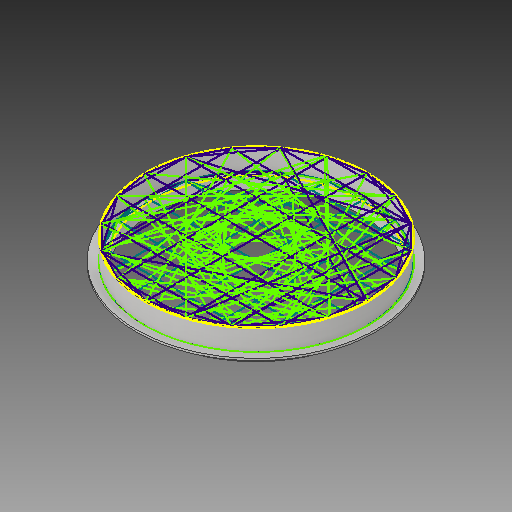
# Autodesk Inventor part: 除沫器
Saved by Autodesk Inventor 2018.2 (Build 222227000, 227)
## iProperties
Created: 2018-07-04
Part Number: 除沫器
Material: 常规
Document SubType Name: Modeling
Designer: Administrator
Density: 1 g/cm^3
Appearance: 默认
Author: Administrator
Autodesk Inventor part; units mm, degrees
ref_plane "YZ Plane" through (0, 0, 0) normal (1, 0, 0) x (0, 1, 0)
ref_plane "XZ Plane" through (0, 0, 0) normal (0, 1, 0) x (-1, 0, 0)
ref_plane "XY Plane" through (0, 0, 0) normal (0, 0, 1) x (1, 0, 0)
sketch "草图1" plane through (0, 0, 0) normal (0, 1, 0) x (-1, 0, 0)
  circle A0 centre (0, 0) radius 575
  circle A1 centre (0, 0) radius 510
  dimension "d0" = 1150
  dimension "d1" = 1020
  constraints: 2 centre point, 2 coincident
  measures "d0" diameter of A0
  measures "d1" diameter of A1
extrude "拉伸1" add sketch "草图1" along normal blind 10
sketch "草图2" plane through (0, 0, 0) normal (0, 1, 0) x (-1, 0, 0)
  circle A0 centre (0, 0) radius 510 projected
surface extrude "拉伸曲面1" sketch "草图2" along normal blind 10 and the other way blind 50 shown no curves A0
thicken "加厚1" operation add thickness 5 both sides no extend neighbours no toward (0.7479816, 0, 0.6637194) faces at (-381.4706, 6.6667, -338.4969) (-381.4706, -30, -338.4969)
sketch "草图3" plane through (0, 10, 0) normal (0, 1, 0) x (1, 0, 0)
  circle A0 centre (0, 0) radius 575 projected
  circle A1 centre (0, 0) radius 536.0493
  constraints: 1 centre point, 1 coincident
surface extrude "拉伸曲面2" sketch "草图3" along normal blind 100 shown no curves A1
thicken "加厚2" operation add thickness 5 both sides no extend neighbours no toward (-0.9991732, 0, -0.0406567) faces at (535.606, 76.6667, 21.794)
sketch "草图4" plane through (0, 110, 0) normal (0, 1, 0) x (1, 0, 0)
  circle A0 centre (0, 0) radius 536.0493 projected
  circle A1 centre (0, 0) radius 531.0493 projected
  line L0 (531.0493, 0) -> (505.0579, -164.1032)
  line L1 (505.0579, -164.1032) -> (429.6279, -312.1429)
  line L2 (429.6279, -312.1429) -> (312.1429, -429.6279)
  line L3 (312.1429, -429.6279) -> (164.1032, -505.0579)
  line L4 (164.1032, -505.0579) -> (0, -531.0493)
  line L5 (0, -531.0493) -> (-164.1032, -505.0579)
  line L6 (-164.1032, -505.0579) -> (-312.1429, -429.6279)
  line L7 (-312.1429, -429.6279) -> (-429.6279, -312.1429)
  line L8 (-429.6279, -312.1429) -> (-505.0579, -164.1032)
  line L9 (-505.0579, -164.1032) -> (-531.0493, 0)
  line L10 (-531.0493, 0) -> (-505.0579, 164.1032)
  line L11 (-505.0579, 164.1032) -> (-429.6279, 312.1429)
  line L12 (-429.6279, 312.1429) -> (-312.1429, 429.6279)
  line L13 (-312.1429, 429.6279) -> (-164.1032, 505.0579)
  line L14 (-164.1032, 505.0579) -> (0, 531.0493)
  line L15 (0, 531.0493) -> (164.1032, 505.0579)
  line L16 (164.1032, 505.0579) -> (312.1429, 429.6279)
  line L17 (312.1429, 429.6279) -> (429.6279, 312.1429)
  line L18 (429.6279, 312.1429) -> (505.0579, 164.1032)
  line L19 (505.0579, 164.1032) -> (531.0493, 0)
  line L20 (-531.0493, 0) -> (531.0493, 0)
  line L21 (-505.0579, 164.1032) -> (-505.0579, -164.1032)
  line L22 (-429.6279, 312.1429) -> (-429.6279, -312.1429)
  line L23 (-312.1429, 429.6279) -> (-312.1429, -429.6279)
  line L24 (-164.1032, 505.0579) -> (-164.1032, -505.0579)
  line L25 (0, 531.0493) -> (0, -531.0493)
  line L26 (164.1032, 505.0579) -> (164.1032, -505.0579)
  line L27 (312.1429, -429.6279) -> (312.1429, 429.6279)
  line L28 (429.6279, 312.1429) -> (429.6279, -312.1429)
  line L29 (505.0579, -164.1032) -> (505.0579, 164.1032)
  line L30 (-164.1032, 505.0579) -> (164.1032, 505.0579)
  line L31 (312.1429, 429.6279) -> (-312.1429, 429.6279)
  line L32 (-429.6279, 312.1429) -> (429.6279, 312.1429)
  line L33 (505.0579, 164.1032) -> (-505.0579, 164.1032)
  line L34 (-505.0579, -164.1032) -> (505.0579, -164.1032)
  line L35 (-429.6279, -312.1429) -> (429.6279, -312.1429)
  line L36 (312.1429, -429.6279) -> (-312.1429, -435.7931)
  line L37 (-164.1032, -505.0579) -> (164.1032, -505.0579)
  line L38 (-312.1429, 429.6279) -> (-505.0579, 164.1032)
  line L39 (-505.0579, -164.1032) -> (-312.1429, -435.7931)
  line L40 (0, -531.0493) -> (-312.1429, -435.7931)
  line L41 (0, -531.0493) -> (312.1429, -429.6279)
  line L42 (312.1429, -429.6279) -> (505.0579, -164.1032)
  line L43 (505.0579, 164.1032) -> (312.1429, 429.6279)
  line L44 (312.1429, 429.6279) -> (0, 531.0493)
  line L45 (531.0493, 0) -> (-312.1429, -435.7931)
  line L46 (-312.1429, 429.6279) -> (531.0493, 0)
  line L47 (312.1429, 429.6279) -> (164.1032, -505.0579)
  line L48 (164.1032, -505.0579) -> (-505.0579, 164.1032)
  line L49 (-505.0579, 164.1032) -> (312.1429, 429.6279)
  line L50 (-429.6279, -312.1429) -> (429.6279, -312.1429)
  line L51 (0, 531.0493) -> (435.7931, -312.1429)
  line L52 (-429.6279, -312.1429) -> (0, 531.0493)
  line L53 (-312.1429, -429.6279) -> (505.0579, -164.1032)
  line L54 (-312.1429, -429.6279) -> (-164.1032, 505.0579)
  line L55 (-164.1032, 505.0579) -> (510.9213, -162.1981)
  line L56 (-505.9804, -165.9401) -> (161.2755, 509.0845)
  line L57 (428.7053, -313.9798) -> (-505.9804, -165.9401)
  line L58 (429.6279, -312.1429) -> (164.1032, 505.0579)
  line L59 (164.1032, -505.0579) -> (-505.0579, 164.1032)
  line L60 (-505.0579, 164.1032) -> (431.533, 318.0064)
  line L61 (164.1032, -505.0579) -> (429.6279, 312.1429)
  line L62 (-429.6279, 312.1429) -> (508.6817, 169.091)
  line L63 (0, -531.0493) -> (-429.6279, 312.1429)
  line L64 (0, -531.0493) -> (505.0579, 164.1032)
  line L65 (311.2203, -431.4647) -> (-536.9596, -5.4607)
  line L66 (164.1032, 505.0579) -> (-531.0493, 0)
  line L67 (163.1807, 503.221) -> (311.2203, -431.4647)
  line L68 (-316.3703, 426.5245) -> (535.9751, 8.9171)
  line L69 (-159.1077, -506.6538) -> (531.0234, 5.2442)
  line L70 (-159.1077, -506.6538) -> (-316.3703, 426.5245)
  line L71 (508.2003, -154.0967) -> (-425.1685, -326.4668)
  line L72 (-174.0458, 501.7184) -> (508.2003, -154.0967)
  line L73 (-174.0458, 501.7184) -> (-423.3795, -320.5669)
  line L74 (-111.947, 217.7208) -> (244.5252, -11.9114)
  line L75 (244.5252, -11.9114) -> (-132.5782, -205.8094)
  line L76 (-132.5782, -205.8094) -> (-111.947, 217.7208)
  line L77 (-210.9866, 63.9755) -> (160.8977, 150.7321)
  line L78 (160.8977, 150.7321) -> (50.0889, -214.7075)
  line L79 (50.0889, -214.7075) -> (-210.9866, 63.9755)
  line L80 (-231.596, -76.5164) -> (49.5329, 238.8263)
  line L81 (49.5329, 238.8263) -> (182.0632, -162.3098)
  line L82 (182.0632, -162.3098) -> (-231.596, -76.5164)
  line L83 (-178.3739, -185.5628) -> (-71.5151, 247.2577)
  line L84 (-71.5151, 247.2577) -> (249.889, -61.6949)
  line L85 (249.889, -61.6949) -> (-178.3739, -185.5628)
  line L86 (-84.545, -232.6889) -> (-159.242, 189.5626)
  line L87 (-159.242, 189.5626) -> (243.787, 43.1263)
  line L88 (243.787, 43.1263) -> (-84.545, -232.6889)
  line L89 (0, -247.9487) -> (-214.7299, 123.9744)
  line L90 (-214.7299, 123.9744) -> (214.7299, 123.9744)
  line L91 (214.7299, 123.9744) -> (0, -247.9487)
  line L92 (79.8324, -233.2057) -> (-241.8782, 47.466)
  line L93 (-241.8782, 47.466) -> (162.0458, 185.7397)
  line L94 (162.0458, 185.7397) -> (79.8324, -233.2057)
  line L95 (218.5126, -161.5306) -> (-249.1459, -108.4722)
  line L96 (-249.1459, -108.4722) -> (30.6333, 270.0028)
  line L97 (30.6333, 270.0028) -> (218.5126, -161.5306)
  point P0 (0, 0)
  point P1 (0, 0)
  point P2 (0, 0)
  point P3 (0, 0)
  constraints: 196 end point, 15 point on line, 13 parallel, 7 coincident, 2 midpoint, 2 perpendicular, 2 point on circle, 1 horizontal, 99 other
sketch "草图5" plane through (0, 10, 0) normal (0, 1, 0) x (1, 0, 0)
  circle A0 centre (0, 0) radius 531.0493 projected
  circle A1 centre (0, 0) radius 505 projected
  circle A2 centre (0, 0) radius 536.0493
  circle A3 centre (0, 0) radius 531.0493
  line L0 (531.0493, 0) -> (505.0579, -164.1032)
  line L1 (505.0579, -164.1032) -> (429.6279, -312.1429)
  line L2 (429.6279, -312.1429) -> (312.1429, -429.6279)
  line L3 (312.1429, -429.6279) -> (164.1032, -505.0579)
  line L4 (164.1032, -505.0579) -> (0, -531.0493)
  line L5 (0, -531.0493) -> (-164.1032, -505.0579)
  line L6 (-164.1032, -505.0579) -> (-312.1429, -429.6279)
  line L7 (-312.1429, -429.6279) -> (-429.6279, -312.1429)
  line L8 (-429.6279, -312.1429) -> (-505.0579, -164.1032)
  line L9 (-505.0579, -164.1032) -> (-531.0493, 0)
  line L10 (-531.0493, 0) -> (-505.0579, 164.1032)
  line L11 (-505.0579, 164.1032) -> (-429.6279, 312.1429)
  line L12 (-429.6279, 312.1429) -> (-312.1429, 429.6279)
  line L13 (-312.1429, 429.6279) -> (-164.1032, 505.0579)
  line L14 (-164.1032, 505.0579) -> (0, 531.0493)
  line L15 (0, 531.0493) -> (164.1032, 505.0579)
  line L16 (164.1032, 505.0579) -> (312.1429, 429.6279)
  line L17 (312.1429, 429.6279) -> (429.6279, 312.1429)
  line L18 (429.6279, 312.1429) -> (505.0579, 164.1032)
  line L19 (505.0579, 164.1032) -> (531.0493, 0)
  line L20 (-531.0493, 0) -> (531.0493, 0)
  line L21 (-505.0579, 164.1032) -> (-505.0579, -164.1032)
  line L22 (-429.6279, 312.1429) -> (-429.6279, -312.1429)
  line L23 (-312.1429, 429.6279) -> (-312.1429, -429.6279)
  line L24 (-164.1032, 505.0579) -> (-164.1032, -505.0579)
  line L25 (0, 531.0493) -> (0, -531.0493)
  line L26 (164.1032, 505.0579) -> (164.1032, -505.0579)
  line L27 (312.1429, -429.6279) -> (312.1429, 429.6279)
  line L28 (429.6279, 312.1429) -> (429.6279, -312.1429)
  line L29 (505.0579, -164.1032) -> (505.0579, 164.1032)
  line L30 (-164.1032, 505.0579) -> (164.1032, 505.0579)
  line L31 (312.1429, 429.6279) -> (-312.1429, 429.6279)
  line L32 (-429.6279, 312.1429) -> (429.6279, 312.1429)
  line L33 (505.0579, 164.1032) -> (-505.0579, 164.1032)
  line L34 (-505.0579, -164.1032) -> (505.0579, -164.1032)
  line L35 (-429.6279, -312.1429) -> (429.6279, -312.1429)
  line L36 (312.1429, -429.6279) -> (-312.1429, -435.7931)
  line L37 (-164.1032, -505.0579) -> (164.1032, -505.0579)
  line L38 (-312.1429, 429.6279) -> (-505.0579, 164.1032)
  line L39 (-505.0579, -164.1032) -> (-312.1429, -435.7931)
  line L40 (0, -531.0493) -> (-312.1429, -435.7931)
  line L41 (0, -531.0493) -> (312.1429, -429.6279)
  line L42 (312.1429, -429.6279) -> (505.0579, -164.1032)
  line L43 (505.0579, 164.1032) -> (312.1429, 429.6279)
  line L44 (312.1429, 429.6279) -> (0, 531.0493)
  line L45 (531.0493, 0) -> (-312.1429, -435.7931)
  line L46 (-312.1429, 429.6279) -> (531.0493, 0)
  line L47 (312.1429, 429.6279) -> (164.1032, -505.0579)
  line L48 (164.1032, -505.0579) -> (-505.0579, 164.1032)
  line L49 (-505.0579, 164.1032) -> (312.1429, 429.6279)
  line L50 (-429.6279, -312.1429) -> (429.6279, -312.1429)
  line L51 (-429.6279, -312.1429) -> (0, 531.0493)
  line L52 (0, 531.0493) -> (435.7931, -312.1429)
  line L53 (-164.1032, 505.0579) -> (510.9213, -162.1981)
  line L54 (-312.1429, -429.6279) -> (-164.1032, 505.0579)
  line L55 (-312.1429, -429.6279) -> (505.0579, -164.1032)
  line L56 (428.7053, -313.9798) -> (-505.9804, -165.9401)
  line L57 (-505.9804, -165.9401) -> (161.2755, 509.0845)
  line L58 (429.6279, -312.1429) -> (164.1032, 505.0579)
  line L59 (-505.0579, 164.1032) -> (431.533, 318.0064)
  line L60 (164.1032, -505.0579) -> (-505.0579, 164.1032)
  line L61 (164.1032, -505.0579) -> (429.6279, 312.1429)
  line L62 (-429.6279, 312.1429) -> (508.6817, 169.091)
  line L63 (0, -531.0493) -> (505.0579, 164.1032)
  line L64 (0, -531.0493) -> (-429.6279, 312.1429)
  line L65 (311.2203, -431.4647) -> (-536.9596, -5.4607)
  line L66 (164.1032, 505.0579) -> (-531.0493, 0)
  line L67 (163.1807, 503.221) -> (311.2203, -431.4647)
  line L68 (-316.3703, 426.5245) -> (535.9751, 8.9171)
  line L69 (-159.1077, -506.6538) -> (-316.3703, 426.5245)
  line L70 (-159.1077, -506.6538) -> (531.0234, 5.2442)
  line L71 (-174.0458, 501.7184) -> (-423.3795, -320.5669)
  line L72 (-174.0458, 501.7184) -> (508.2003, -154.0967)
  line L73 (508.2003, -154.0967) -> (-425.1685, -326.4668)
  line L74 (-111.947, 217.7208) -> (244.5252, -11.9114)
  line L75 (244.5252, -11.9114) -> (-132.5782, -205.8094)
  line L76 (-132.5782, -205.8094) -> (-111.947, 217.7208)
  line L77 (-210.9866, 63.9755) -> (160.8977, 150.7321)
  line L78 (160.8977, 150.7321) -> (50.0889, -214.7075)
  line L79 (50.0889, -214.7075) -> (-210.9866, 63.9755)
  line L80 (-231.596, -76.5164) -> (49.5329, 238.8263)
  line L81 (49.5329, 238.8263) -> (182.0632, -162.3098)
  line L82 (182.0632, -162.3098) -> (-231.596, -76.5164)
  line L83 (-178.3739, -185.5628) -> (-71.5151, 247.2577)
  line L84 (-71.5151, 247.2577) -> (249.889, -61.6949)
  line L85 (249.889, -61.6949) -> (-178.3739, -185.5628)
  line L86 (-84.545, -232.6889) -> (-159.242, 189.5626)
  line L87 (-159.242, 189.5626) -> (243.787, 43.1263)
  line L88 (243.787, 43.1263) -> (-84.545, -232.6889)
  line L89 (0, -247.9487) -> (-214.7299, 123.9744)
  line L90 (-214.7299, 123.9744) -> (214.7299, 123.9744)
  line L91 (214.7299, 123.9744) -> (0, -247.9487)
  line L92 (79.8324, -233.2057) -> (-241.8782, 47.466)
  line L93 (-241.8782, 47.466) -> (162.0458, 185.7397)
  line L94 (162.0458, 185.7397) -> (79.8324, -233.2057)
  line L95 (218.5126, -161.5306) -> (-249.1459, -108.4722)
  line L96 (-249.1459, -108.4722) -> (30.6333, 270.0028)
  line L97 (30.6333, 270.0028) -> (218.5126, -161.5306)
  point P0 (0, 0)
  point P1 (0, 0)
  point P2 (0, 0)
  point P3 (0, 0)
  constraints: 196 end point, 15 point on line, 13 parallel, 7 coincident, 2 midpoint, 2 perpendicular, 2 point on circle, 1 centre point, 1 horizontal, 100 other
body "Srf1"
body "Srf2"
